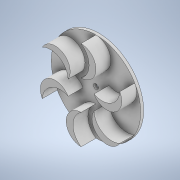
# Autodesk Inventor part: 20220606_ファン
Saved by Autodesk Inventor 2020 (Build 240168000, 168)
## iProperties
Created: 2022-06-06
Part Number: 20220606_ファン
Material: 一般
Document SubType Name: Modeling
Designer: Naggy
Density: 1 g/cm^3
Appearance: 既定
Author: Naggy
Autodesk Inventor part; units mm, degrees
ref_plane "YZ Plane" through (0, 0, 0) normal (1, 0, 0) x (0, 1, 0)
ref_plane "XZ Plane" through (0, 0, 0) normal (0, 1, 0) x (-1, 0, 0)
ref_plane "XY Plane" through (0, 0, 0) normal (0, 0, 1) x (1, 0, 0)
sketch "スケッチ1" plane through (0, 0, 0) normal (0, 0, 1) x (1, 0, 0)
  circle A0 centre (0, 0) radius 15
  dimension "d0" = 30
  constraints: 1 centre point, 1 coincident
  measures "d0" diameter of A0
extrude "押し出し1" add sketch "スケッチ1" along normal blind 1
sketch "スケッチ2" plane through (0, 0, 1) normal (0, 0, 1) x (1, 0, 0)
  circle A0 centre (0, 0) radius 5
  circle A1 centre (0, 0) radius 15 projected
  arc A2 (0, 5) -> (0, 15) centre (0, 10) ccw
  arc A3 (0, 5) -> (0, 15) centre (-3.3, 10) ccw
  arc A4 (-4.3301, 2.5) -> (-12.9904, 7.5) centre (-8.6603, 5) ccw
  arc A5 (-4.3301, 2.5) -> (-12.9904, 7.5) centre (-10.3103, 2.1421) ccw
  arc A6 (-4.3301, -2.5) -> (-12.9904, -7.5) centre (-8.6603, -5) ccw
  arc A7 (-4.3301, -2.5) -> (-12.9904, -7.5) centre (-7.0103, -7.8579) ccw
  arc A8 (0, -5) -> (0, -15) centre (0, -10) ccw
  arc A9 (0, -5) -> (0, -15) centre (3.3, -10) ccw
  arc A10 (4.3301, -2.5) -> (12.9904, -7.5) centre (8.6603, -5) ccw
  arc A11 (4.3301, -2.5) -> (12.9904, -7.5) centre (10.3103, -2.1421) ccw
  arc A12 (4.3301, 2.5) -> (12.9904, 7.5) centre (8.6603, 5) ccw
  arc A13 (4.3301, 2.5) -> (12.9904, 7.5) centre (7.0103, 7.8579) ccw
  dimension "d3" = 10
  dimension "d4" = 3.3
  dimension "d7" = 360
  constraints: 24 point on circle, 12 centre point, 2 vertical alignment, 1 coincident, 41 other
  measures "d4" distance of A2.centre A3.centre
extrude "押し出し2" add sketch "スケッチ2" along normal blind 5 contours A13 A12 | A11 A10 | A3 A2 | A9 A8 | A5 A4 | A7 A6
sketch "スケッチ3" plane through (0, 0, 1) normal (0, 0, 1) x (1, 0, 0)
  point P0 (0, 0)
  point P1 (0, 0)
  constraints: 1 coincident
hole "穴1" at (0, 0, 1) direction (0, 0, -1) diameter 1.7 depth 8.8 tip angle 118
